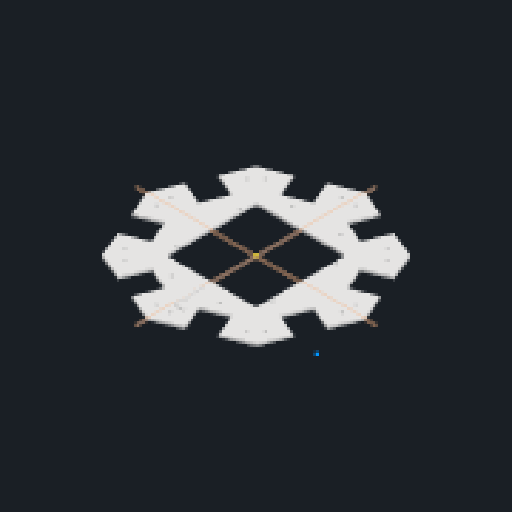
# Autodesk Inventor part: Bund
Saved by Autodesk Inventor 2026.2 (Build 302298000, 298)
## iProperties
Created: 2026-04-22
Part Number: Bund
Material: Generic
Document SubType Name: Modeling
Designer: Mikke
Density: 1 g/cm^3
Appearance: Default
Author: Mikke
Autodesk Inventor part; units mm, degrees
ref_plane "YZ Plane" through (0, 0, 0) normal (1, 0, 0) x (0, 1, 0)
ref_plane "XZ Plane" through (0, 0, 0) normal (0, 1, 0) x (-1, 0, 0)
ref_plane "XY Plane" through (0, 0, 0) normal (0, 0, 1) x (1, 0, 0)
sketch "Sketch1" plane through (0, 0, 0) normal (0, 1, 0) x (-1, 0, 0)
  line L0 (0, 0) -> (0, -104.6)
  line L1 (0, -104.6) -> (-73.9634, -73.9634)
  line L2 (-73.9634, -73.9634) -> (-104.6, 0)
  line L3 (-104.6, 0) -> (-73.9634, 73.9634)
  line L4 (-73.9634, 73.9634) -> (0, 104.6)
  line L5 (0, 104.6) -> (73.9634, 73.9634)
  line L6 (73.9634, 73.9634) -> (104.6, 0)
  line L7 (104.6, 0) -> (73.9634, -73.9634)
  line L8 (73.9634, -73.9634) -> (0, -104.6)
  line L9 (89.2707, -89.2707) -> (126.2478, 0)
  line L10 (126.2478, 0) -> (89.2707, 89.2707)
  line L11 (89.2707, 89.2707) -> (0, 126.2478)
  line L12 (0, 126.2478) -> (-89.2707, 89.2707)
  line L13 (-89.2707, 89.2707) -> (-126.2478, 0)
  line L14 (-126.2478, 0) -> (-89.2707, -89.2707)
  line L15 (-89.2707, -89.2707) -> (0, -126.2478)
  line L16 (0, -126.2478) -> (89.2707, -89.2707)
  line L17 (0, -104.6) -> (7.6537, -123.0776)
  line L18 (0, -104.6) -> (20, -104.6) construction
  line L19 (73.9634, -73.9634) -> (81.617, -92.441)
  line L20 (73.9634, -73.9634) -> (76.2595, -79.5066)
  line L21 (76.2595, -79.5066) -> (70.7162, -81.8027)
  circle A0 centre (70.7162, -81.8027) radius 1.6
  line L22 (0, -104.6) -> (2.2961, -110.1433)
  line L23 (2.2961, -110.1433) -> (7.8394, -107.8472)
  circle A1 centre (7.8394, -107.8472) radius 1.6
  circle A2 centre (107.8472, -7.8394) radius 1.6
  circle A3 centre (81.8027, -70.7162) radius 1.6
  circle A4 centre (81.8027, 70.7162) radius 1.6
  circle A5 centre (107.8472, 7.8394) radius 1.6
  circle A6 centre (7.8394, 107.8472) radius 1.6
  circle A7 centre (70.7162, 81.8027) radius 1.6
  circle A8 centre (-70.7162, 81.8027) radius 1.6
  circle A9 centre (-7.8394, 107.8472) radius 1.6
  circle A10 centre (-107.8472, 7.8394) radius 1.6
  circle A11 centre (-81.8027, 70.7162) radius 1.6
  circle A12 centre (-81.8027, -70.7162) radius 1.6
  circle A13 centre (-107.8472, -7.8394) radius 1.6
  circle A14 centre (-7.8394, -107.8472) radius 1.6
  circle A15 centre (-70.7162, -81.8027) radius 1.6
  dimension "d0" = 104.6
  dimension "d1" = 20
  dimension "d2" = 67.5
  dimension "d3" = 6
  dimension "d4" = 6
  dimension "d5" = 3.2
  dimension "d6" = 6
  dimension "d7" = 3.2
  dimension "d10" = 360
  constraints: 48 end point, 16 centre point, 4 point on line, 3 coincident, 3 perpendicular, 1 equal length, 1 horizontal, 1 vertical, 57 other
  measures "d0" distance of L0.start L0.end
  measures "d1" distance between parallel lines of L7 L9
  measures "d2" angle of L17 L18
  measures "d3" distance of L7.end L20.end
  measures "d4" distance of L20.end L21.end
  measures "d5" diameter of A0
  measures "d6" distance of L22.end L23.end
  measures "d7" diameter of A1
extrude "Extrusion1" add sketch "Sketch1" along normal blind 3
ref_plane "Work Plane1" through (126.2478, 0, 0) normal (0, 0, 1) x (0, 1, 0)
ref_plane "Work Plane2" through (0, 0, -126.2478) normal (1, 0, 0) x (0, 1, 0)
sketch "Sketch3" plane through (0, 0, 0) normal (0, -1, 0) x (1, 0, 0)
  line L0 (-49.9941, -52.4) -> (49.9941, -52.4) construction
  line L1 (49.9941, -52.4) -> (52.4, -49.9941) construction
  line L2 (52.4, -49.9941) -> (52.4, 49.9941) construction
  line L3 (52.4, 49.9941) -> (49.9941, 52.4) construction
  line L4 (49.9941, 52.4) -> (-49.9941, 52.4) construction
  line L5 (-49.9941, 52.4) -> (-52.4, 49.9941) construction
  line L6 (-52.4, 49.9941) -> (-52.4, -49.9941) construction
  line L7 (-52.4, -49.9941) -> (-49.9941, -52.4) construction
  circle A0 centre (-45, -45) radius 1.25 construction
  circle A1 centre (44.8952, -45.0207) radius 1.25 construction
  circle A2 centre (45.9242, 45.9242) radius 1.25 construction
  line L8 (-50.077, 52.6) -> (50.077, 52.6)
  line L9 (50.077, 52.6) -> (52.6, 50.077)
  line L10 (52.6, 50.077) -> (52.6, -50.077)
  line L11 (52.6, -50.077) -> (50.077, -52.6)
  line L12 (50.077, -52.6) -> (-50.077, -52.6)
  line L13 (-50.077, -52.6) -> (-52.6, -50.077)
  line L14 (-52.6, -50.077) -> (-52.6, 50.077)
  line L15 (-52.6, 50.077) -> (-50.077, 52.6)
  point P0 (0, 0)
  dimension "d24" = 0.2
  constraints: 16 end point, 7 other
  measures "d24" distance between parallel lines of L4 L8
extrude "Extrusion3" cut sketch "Sketch3" against normal through all
sketch "Sketch4" plane through (0, 3, 0) normal (0, 1, 0) x (1, 0, 0)
  circle A0 centre (55.9, -37.4) radius 1.75 projected
  circle A1 centre (55.9, 37.4) radius 1.75 projected
  circle A2 centre (-55.9, 37.4) radius 1.75 projected
  circle A3 centre (-55.9, -37.4) radius 1.75 projected
  point P0 (0, 0)
extrude "Extrusion4" cut sketch "Sketch4" against normal blind 10
sketch "Sketch6" plane through (0, 3, 0) normal (0, 1, 0) x (1, 0, 0)
  line L0 (0, 0) -> (-44.6354, -107.7593) construction
  line L1 (-89.2707, -89.2707) -> (0, -126.2478) projected
  line L2 (-33.5487, -120.1907) -> (-19.2967, -85.7831)
  line L3 (-19.2967, -85.7831) -> (-47.013, -74.3026)
  line L4 (-47.013, -74.3026) -> (-61.2651, -108.7102)
  line L5 (-61.2651, -108.7102) -> (-33.5487, -120.1907)
  line L6 (-33.5487, -120.1907) -> (-47.013, -74.3026) construction
  line L7 (-19.2967, -85.7831) -> (-61.2651, -108.7102) construction
  point P0 (-40.2809, -97.2467)
  point P1 (-58.4935, -102.019)
  point P2 (-30.7772, -113.4995)
  dimension "d34" = 30
  dimension "d35" = 30
  constraints: 14 end point, 3 midpoint, 2 parallel, 1 perpendicular, 1 point on line
  measures "d34" distance between parallel lines of L1 L3
  measures "d35" distance between parallel lines of L2 L4
extrude "Extrusion6" cut sketch "Sketch6" against normal blind 10 contours L4 L3 L2 L1
pattern_circular "Circular Pattern1" count 8 over 360 about axis through (0, -10, 0) along (0, 1, 0) of "Extrusion6"
sketch "Sketch7" plane through (0, 3, 0) normal (0, 1, 0) x (1, 0, 0)
  circle A0 centre (-28, -70) radius 1.75
  circle A1 centre (-28, 70) radius 1.75
  line L0 (0, 176.747) -> (0, -176.747) projected
  line L1 (-30.7772, -113.4995) -> (0, -126.2478) projected
  line L2 (0, 126.2478) -> (-30.7772, 113.4995) projected
  line L3 (0, -126.2478) -> (0, 126.2478)
  circle A2 centre (28, -70) radius 1.75
  circle A3 centre (28, 70) radius 1.75
  point P0 (0, 0)
  dimension "d41" = 3.5
  dimension "d42" = 3.5
  dimension "d43" = 70
  dimension "d44" = 70
  dimension "d45" = 28
  dimension "d46" = 28
  constraints: 4 centre point, 2 end point, 2 symmetric about line, 1 vertical, 2 other
  measures "d41" diameter of A0
  measures "d42" diameter of A1
  measures "d43" vertical distance of point (0, 0) A0.centre
  measures "d44" vertical distance of A1.centre point (0, 0)
  measures "d45" horizontal distance of point (0, 0) A0.centre
  measures "d46" distance from line of L0 A1.centre
extrude "Extrusion7" cut sketch "Sketch7" against normal blind 10
sketch "Sketch8" plane through (0, 3, 0) normal (0, 1, 0) x (1, 0, 0)
  line L0 (3, -87.2498) -> (-3, -87.2498)
  line L1 (-3, -87.2498) -> (-3, -62.8198)
  line L2 (-3, -62.8198) -> (3, -62.8198)
  line L3 (3, -62.8198) -> (3, -87.2498)
  line L4 (0, 176.747) -> (0, -176.747) projected
  line L5 (5.7649, -85.1044) -> (0, -85.1044)
  line L6 (0, -96.9388) -> (5.7649, -85.1044)
  line L7 (-5.7649, -85.1044) -> (0, -85.1044)
  line L8 (0, -96.9388) -> (-5.7649, -85.1044)
  line L9 (15.0282, -98.8586) -> (0.1461, -98.8586) construction
  line L10 (0.1461, -98.8586) -> (0.1461, -93.7303) construction
  line L11 (0.1461, -93.7303) -> (15.0282, -93.7303) construction
  line L12 (15.0282, -93.7303) -> (15.0282, -98.8586) construction
  line L13 (12.1012, -95.7464) -> (12.8373, -95.7464)
  line L14 (12.8373, -95.7464) -> (14.013, -97.8706)
  line L15 (14.013, -97.8706) -> (14.013, -95.7464)
  line L16 (14.013, -95.7464) -> (14.712, -95.7464)
  line L17 (14.712, -95.7464) -> (14.712, -98.7944)
  line L18 (14.712, -98.7944) -> (13.7734, -98.7944)
  line L19 (13.7734, -98.7944) -> (12.8002, -97.0481)
  line L20 (12.8002, -97.0481) -> (12.8002, -98.7944)
  line L21 (12.8002, -98.7944) -> (12.1012, -98.7944)
  line L22 (12.1012, -98.7944) -> (12.1012, -95.7464)
  spline S0 degree 2 poles (8.7074, -97.2704) (8.7074, -96.5294) (9.4978, -95.6822) (10.1845, -95.6822) knots 0 0 0 1 2 2 2
  spline S1 degree 2 poles (10.1845, -95.6822) (10.8736, -95.6822) (11.6591, -96.5393) (11.6591, -97.2704) knots 0 0 0 1 2 2 2
  spline S2 degree 2 poles (11.6591, -97.2704) (11.6591, -98.004) (10.8736, -98.8586) (10.1845, -98.8586) knots 0 0 0 1 2 2 2
  spline S3 degree 2 poles (10.1845, -98.8586) (9.4978, -98.8586) (8.7074, -98.009) (8.7074, -97.2704) knots 0 0 0 1 2 2 2
  spline S4 degree 2 poles (9.4978, -97.2704) (9.4978, -97.5446) (9.6089, -97.9274) (9.7053, -98.0485) knots 0 0 0 1 2 2 2
  spline S5 degree 2 poles (9.7053, -98.0485) (9.8016, -98.1744) (10.0486, -98.2831) (10.182, -98.2831) knots 0 0 0 1 2 2 2
  spline S6 degree 2 poles (10.182, -98.2831) (10.3228, -98.2831) (10.5525, -98.1819) (10.6587, -98.0534) knots 0 0 0 1 2 2 2
  spline S7 degree 2 poles (10.6587, -98.0534) (10.7526, -97.9349) (10.8687, -97.5421) (10.8687, -97.2704) knots 0 0 0 1 2 2 2
  spline S8 degree 2 poles (10.8687, -97.2704) (10.8687, -96.9888) (10.7575, -96.6183) (10.6612, -96.4924) knots 0 0 0 1 2 2 2
  spline S9 degree 2 poles (10.6612, -96.4924) (10.5648, -96.3664) (10.3154, -96.2577) (10.182, -96.2577) knots 0 0 0 1 2 2 2
  spline S10 degree 2 poles (10.182, -96.2577) (10.0461, -96.2577) (9.7942, -96.3738) (9.7028, -96.4973) knots 0 0 0 1 2 2 2
  spline S11 degree 2 poles (9.7028, -96.4973) (9.604, -96.6307) (9.4978, -96.9839) (9.4978, -97.2704) knots 0 0 0 1 2 2 2
  line L23 (5.4371, -95.7464) -> (6.3683, -95.7464)
  line L24 (6.3683, -95.7464) -> (7.2155, -96.8653)
  line L25 (7.2155, -96.8653) -> (7.4921, -96.8653)
  line L26 (7.4921, -96.8653) -> (7.4921, -95.7464)
  line L27 (7.4921, -95.7464) -> (8.2529, -95.7464)
  line L28 (8.2529, -95.7464) -> (8.2529, -98.7944)
  line L29 (8.2529, -98.7944) -> (7.0278, -98.7944)
  spline S12 degree 2 poles (7.0278, -98.7944) (6.7734, -98.7944) (6.3979, -98.7302) (6.2374, -98.6314) knots 0 0 0 1 2 2 2
  spline S13 degree 2 poles (6.2374, -98.6314) (6.0743, -98.5277) (5.8817, -98.2041) (5.8817, -97.9571) knots 0 0 0 1 2 2 2
  spline S14 degree 2 poles (5.8817, -97.9571) (5.8817, -97.6088) (6.1978, -97.1716) (6.4621, -97.0432) knots 0 0 0 1 2 2 2
  line L30 (6.4621, -97.0432) -> (5.4371, -95.7464)
  spline S15 degree 2 poles (6.6672, -97.8608) (6.6672, -97.9768) (6.7561, -98.1423) (6.8573, -98.1868) knots 0 0 0 1 2 2 2
  spline S16 degree 2 poles (6.8573, -98.1868) (6.929, -98.2164) (7.1043, -98.2337) (7.2353, -98.2337) knots 0 0 0 1 2 2 2
  line L31 (7.2353, -98.2337) -> (7.4921, -98.2337)
  line L32 (7.4921, -98.2337) -> (7.4921, -97.4137)
  line L33 (7.4921, -97.4137) -> (7.2723, -97.4137)
  spline S17 degree 2 poles (7.2723, -97.4137) (7.1142, -97.4137) (6.8895, -97.4532) (6.8129, -97.5149) knots 0 0 0 1 2 2 2
  spline S18 degree 2 poles (6.8129, -97.5149) (6.7388, -97.5742) (6.6672, -97.7323) (6.6672, -97.8608) knots 0 0 0 1 2 2 2
  spline S19 degree 2 poles (2.4904, -97.2679) (2.4904, -96.8406) (2.8633, -96.1688) (3.1474, -95.9885) knots 0 0 0 1 2 2 2
  spline S20 degree 2 poles (3.1474, -95.9885) (3.3845, -95.8353) (3.9427, -95.7464) (4.2564, -95.7464) knots 0 0 0 1 2 2 2
  line L34 (4.2564, -95.7464) -> (5.2098, -95.7464)
  line L35 (5.2098, -95.7464) -> (5.2098, -98.7944)
  line L36 (5.2098, -98.7944) -> (4.2663, -98.7944)
  spline S21 degree 2 poles (4.2663, -98.7944) (3.9452, -98.7944) (3.3845, -98.7129) (3.1375, -98.5548) knots 0 0 0 1 2 2 2
  spline S22 degree 2 poles (3.1375, -98.5548) (2.8386, -98.3622) (2.4904, -97.7101) (2.4904, -97.2679) knots 0 0 0 1 2 2 2
  spline S23 degree 2 poles (3.2758, -97.2729) (3.2758, -97.5742) (3.4833, -98.004) (3.6957, -98.125) knots 0 0 0 1 2 2 2
  spline S24 degree 2 poles (3.6957, -98.125) (3.8513, -98.209) (4.1922, -98.2263) (4.4293, -98.2263) knots 0 0 0 1 2 2 2
  line L37 (4.4293, -98.2263) -> (4.4441, -98.2263)
  line L38 (4.4441, -98.2263) -> (4.4441, -96.317)
  line L39 (4.4441, -96.317) -> (4.4293, -96.317)
  spline S25 degree 2 poles (4.4293, -96.317) (4.1724, -96.317) (3.8192, -96.3343) (3.6587, -96.4356) knots 0 0 0 1 2 2 2
  spline S26 degree 2 poles (3.6587, -96.4356) (3.471, -96.5541) (3.2758, -96.9715) (3.2758, -97.2729) knots 0 0 0 1 2 2 2
  point P0 (0, 0)
  point P1 (3, -85.1044)
  point P2 (-3, -85.1044)
  dimension "d49" = 3
  dimension "d50" = 6
  constraints: 16 end point, 2 horizontal, 2 parallel, 2 point on line, 1 perpendicular, 1 symmetric about line, 2 other
  measures "d49" distance between parallel lines of L4 L3
  measures "d50" distance between parallel lines of L3 L1
extrude "Extrusion8" add sketch "Sketch8" along normal blind 1
sketch "Sketch9" plane through (0, 3, 0) normal (0, 1, 0) x (1, 0, 0)
  point P0 (0, 0)
ref_plane "Work Plane3" through (107.7593, 0, 44.6354) normal (-0.3827, 0, 0.9239) x (0.9239, 0, 0.3827)
body "Solid1"
